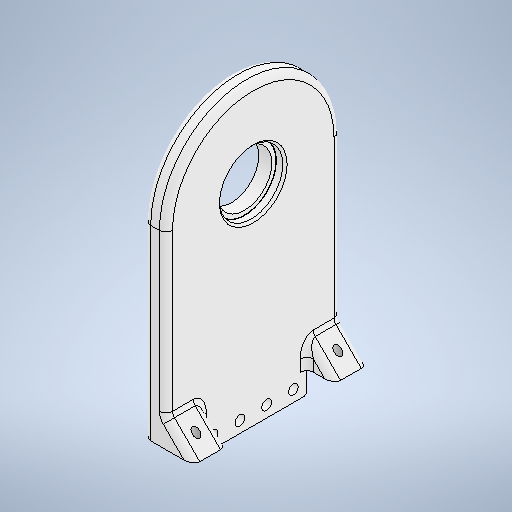
# Autodesk Inventor part: joint4_base_support
Saved by Autodesk Inventor 2025.3 (Build 293356030, 356C)
## iProperties
Created: 2025-11-08
Part Number: joint4_base_support
Material: PLA filament
Document SubType Name: Modeling
Designer: MSI
Density: 1.2 g/cm^3
Appearance: 일반
Mass: 111.315 g
Surface Area: 244.212 cm^2
Volume: 92.7623 cm^3
Author: MSI
Autodesk Inventor part; units mm, degrees
ref_plane "YZ Plane" through (0, 0, 0) normal (1, 0, 0) x (0, 1, 0)
ref_plane "XZ Plane" through (0, 0, 0) normal (0, 1, 0) x (-1, 0, 0)
ref_plane "XY Plane" through (0, 0, 0) normal (0, 0, 1) x (1, 0, 0)
sketch "스케치1" plane through (0, 0, 0) normal (1, 0, 0) x (0, 1, 0)
  circle A0 centre (0, 0) radius 40
  line L0 (0, 40) -> (-96, 40)
  line L1 (-96, 40) -> (-96, -40)
  line L2 (-96, -40) -> (0, -40)
  line L3 (0, -40) -> (0, 40)
  point P0 (0, -40)
  point P1 (0, 40)
  dimension "d0" = 80
  dimension "d1" = 96
  dimension "d2" = 80
  constraints: 8 end point, 2 coincident, 2 parallel, 1 centre point, 1 horizontal, 1 midpoint, 1 perpendicular
  measures "d0" diameter of A0
  measures "d1" distance of L2.end L1.end
  measures "d2" distance of L1.end L0.end
extrude "돌출1" add sketch "스케치1" along normal mid plane 10
sketch "스케치2" plane through (5, 0, 0) normal (1, 0, 0) x (0, 0, -1)
  arc A0 (40, 0) -> (-40, 0) centre (0, 0) ccw projected
  constraints: 1 coincident
hole "구멍1" at (5, 0, 0) direction (-1, 0, 0) diameter 25 end through all counterbore diameter 29 counterbore depth 4
fillet "모깎기1" radius 0.1 1 edges at (1, 0, 14.5)
sketch "스케치3" plane through (-5, -96, 40) normal (0, 0, 1) x (1, 0, 0)
  line L0 (0, 0) -> (10, 0) projected
  line L1 (10, 0) -> (10, 96) projected
  line L2 (0, 0) -> (10, 0)
  line L3 (10, 0) -> (10, 10.5)
  line L4 (10, 10.5) -> (0, 10.5)
  line L5 (0, 10.5) -> (0, 0)
  point P0 (5, 96)
  dimension "d12" = 10.5
  constraints: 8 end point, 2 parallel, 1 horizontal, 1 perpendicular, 1 point on line
  measures "d12" distance between parallel lines of L0 L4
extrude "돌출2" cut sketch "스케치3" against normal blind 15.5
sketch "스케치5" plane through (-5, 0, 40) normal (0, 0, 1) x (1, 0, 0)
  line L0 (10, 0) -> (10, -85.5) projected
  line L1 (10, -73) -> (22.5, -85.5)
  line L2 (22.5, -85.5) -> (10, -85.5)
  point P0 (5, 0)
  dimension "d27" = 45
  dimension "d30" = 12.5
  constraints: 4 end point, 1 horizontal, 1 point on line
  measures "d27" angle of L2 L1
  measures "d30" distance from line of L2 L1.start
extrude "돌출3" add sketch "스케치5" against normal blind 15.5
mirror "미러1" about plane through (0, 0, 0) normal (0, 0, 1) of "돌출2", "돌출3"
sketch "스케치6" plane through (-5, -85.5, 24.5) normal (0, -1, 0) x (1, 0, 0)
  line L0 (5, 8) -> (16.25, 8)
  line L1 (16.25, 8) -> (16.25, -57)
  line L2 (16.25, -57) -> (5, -57)
  line L3 (5, -57) -> (5, 8)
  line L4 (0, 15.5) -> (10, 15.5) projected
  line L5 (22.5, 15.5) -> (10, 15.5) projected
  line L6 (22.5, -64.5) -> (10, -64.5) projected
  line L7 (10, -49) -> (10, -64.5) projected
  line L8 (10, -49) -> (22.5, -49) projected
  line L9 (22.5, -64.5) -> (22.5, -49) projected
  line L10 (22.5, 15.5) -> (10, 15.5) projected
  line L11 (22.5, 15.5) -> (22.5, 0) projected
  line L12 (10, 0) -> (22.5, 0) projected
  line L13 (10, 15.5) -> (10, 0) projected
  point P0 (5, -24.5)
  point P1 (5, 15.5)
  point P2 (16.25, 15.5)
  dimension "d44" = 7.5
  dimension "d45" = 7.5
  constraints: 8 end point, 4 coincident, 2 midpoint, 2 parallel, 2 point on line, 1 horizontal, 1 perpendicular
  measures "d44" distance between parallel lines of L0 L5
  measures "d45" distance between parallel lines of L2 L6
hole "구멍3" at (11.25, -85.5, -32.5) at (0, -85.5, -32.5) at (0, -85.5, 32.5) at (11.25, -85.5, 32.5) direction (0, 1, 0) diameter 3.242 depth 10 tip angle 118 thread size "M4x0.7" class "6H" standard "ISO Metric profile"
sketch "스케치4" plane through (-5, 0, 0) normal (-1, 0, 0) x (0, 0, 1)
  line L0 (-18.375, -90.75) -> (18.375, -90.75)
  line L1 (-24.5, -96) -> (24.5, -96) projected
  line L2 (-24.5, -85.5) -> (-24.5, -96) projected
  point P0 (0, 0)
  point P1 (0, -90.75)
  point P2 (0, -96)
  point P3 (-24.5, -90.75)
  point P4 (-6.125, -90.75)
  point P5 (6.125, -90.75)
  dimension "d17" = 36.75
  dimension "d18" = 12.25
  dimension "d19" = 12.25
  constraints: 3 midpoint, 3 point on line, 2 coincident, 2 end point, 1 horizontal, 1 vertical alignment
  measures "d17" distance of L0.start L0.end
  measures "d18" distance of point (-6.125, -90.75) point (-18.375, -90.75)
  measures "d19" distance of point (6.125, -90.75) point (18.375, -90.75)
hole "구멍2" at (-5, -90.75, -18.375) at (-5, -90.75, -6.125) at (-5, -90.75, 6.125) at (-5, -90.75, 18.375) direction (1, 0, 0) diameter 4.5 end through all counterbore diameter 8 counterbore depth 4.4 clearance for "Socket Head Cap Screw ISO 4762" size "M4" standard "ISO"
fillet "모깎기4" radius 3 2 edges at (11.25, -79.25, 24.5) (11.25, -79.25, -24.5)
fillet "모깎기2" radius 3 4 edges at (0, 0, 40) (0, 0, -40) (5, -73, 33.75) (5, -73, -33.75)
fillet "모깎기3" radius 3 6 edges at (-5, -42.75, -40) (-5, -42.75, 40) (-5, 40, 0) (5, -35.8787, 40) (5, -35.8787, -40) (5, 40, 0)
chamfer "모따기1" distance 1 angle 45 3 edges at (0, -96, 24.5) (0, -96, -24.5) (5, 0, 14.5)
equation "\"d45\" = d44"
equation "\"d17\" = 3 * d18"
equation "\"d19\" = d18"
